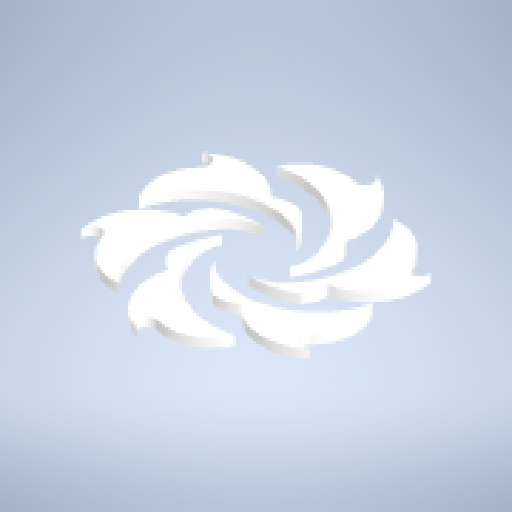
# Autodesk Inventor part: LOGO
Saved by Autodesk Inventor 2026.1 (Build 301233020, 233B)
## iProperties
Created: 2025-07-18
Part Number: LOGO
Material: 一般
Document SubType Name: Modeling
Designer: hibik
Density: 1 g/cm^3
Appearance: 既定
Author: hibik
Autodesk Inventor part; units mm, degrees
ref_plane "YZ Plane" through (0, 0, 0) normal (1, 0, 0) x (0, 1, 0)
ref_plane "XZ Plane" through (0, 0, 0) normal (0, 1, 0) x (-1, 0, 0)
sketch "スケッチ1" plane through (0, 0, 0) normal (0, 1, 0) x (-1, 0, 0)
  circle A0 centre (0, 0) radius 10 construction
  arc A1 (-2.5126, 0.5238) -> (1.9563, -1.6615) centre (0, 0) ccw
  arc A2 (-2.5126, 0.5238) -> (5.8099, -5.8825) centre (3.1979, -0.6667) ccw
  arc A3 (1.9563, -1.6615) -> (5.8099, -5.8825) centre (1.7789, -5.6931) ccw
  arc A4 (0.8333, -8.2275) -> (0.4466, -9.5023) centre (0.6667, -8.873) ccw
  arc A5 (1.9421, -1.6781) -> (4.7391, -6.2927) centre (1.6667, -5) ccw
  arc A6 (-3.2246, -3.3333) -> (-2.633, -0.5) centre (-0.9333, -2.3333) ccw
  arc A7 (-2.3333, -0.2667) -> (-2.3857, -2.355) centre (0.8049, -1.3903) ccw
  arc A8 (-2.3333, -0.2667) -> (-3.2246, -3.3333) centre (2.442, -3.3174) ccw
  point P0 (-2.091, -4.5491)
  point P1 (6.6984, -142.534)
  point P2 (12.5, -123.4123)
  point P3 (71.0869, -94.3908)
  point P4 (-0.885, -4.8329)
  point P5 (-1.6554, -4.7268)
  point P6 (-1.5359, -4.0754)
  point P7 (-39.4956, -7.5004)
  point P8 (87.1485, -88.2381)
  point P9 (1.4768, -1.669)
  point P10 (-1.7561, -3.7466)
  point P11 (1.1339, -1.7095)
  point P12 (1.4776, -1.672)
  point P13 (-2.5333, -0.4124)
  point P14 (-0.5469, -2.5077)
  point P15 (63.4693, -48.0608)
  point P16 (-2.4617, -0.7266)
  point P17 (-2.5059, -0.5553)
  point P18 (-2.6339, -0.7983)
  point P19 (-36.7334, -7.086)
  point P20 (-37.6897, 7.8571)
  point P21 (-35.7696, -6.328)
  point P22 (1.5501, -2.0457)
  point P23 (-0.6623, -2.4798)
  dimension "d0" = 20
  dimension "d1" = 5.1333
  dimension "d7" = 1.3333
  dimension "d9" = 1.6667
  dimension "d10" = 5
  dimension "d11" = 6.6667
  dimension "d13" = 5
  dimension "d15" = 2.3333
  dimension "d16" = 0.9333
  dimension "d17" = 0.6667
  dimension "d18" = 0.6667
  dimension "d19" = 11.6667
  dimension "d20" = 2.3333
  dimension "d21" = 0.2667
  dimension "d23" = 1
  dimension "d24" = 5.6667
  dimension "d25" = 3.3333
  constraints: 22 point on circle, 9 centre point, 6 tangent, 2 coincident
  measures "d0" diameter of A0
  measures "d1" diameter of A1
  measures "d7" diameter of A4
  measures "d9" horizontal distance of point (0, 0) A5.centre
  measures "d10" vertical distance of point (0, 0) A5.centre
  measures "d11" diameter of A5
  measures "d13" diameter of A6
  measures "d15" vertical distance of point (0, 0) A6.centre
  measures "d16" horizontal distance of point (0, 0) A6.centre
  measures "d17" vertical distance of point (0, 0) A2.centre
  measures "d18" horizontal distance of point (0, 0) A4.centre
  measures "d19" diameter of A2
  measures "d20" horizontal distance of point (0, 0) A7.start
  measures "d21" vertical distance of A7.start point (0, 0)
  measures "d23" vertical distance of A6.centre A6.start
  measures "d24" radius of A8
  measures "d25" radius of A7
extrude "押し出し1" add sketch "スケッチ1" along normal blind 0.6667 contours A6 A5 A2 | A2 A5 A6 | A5 A6 A3 A2 | A5 A4 A3 A6 | A8 A7 A1 | A1 A7 A2 A8 | A3 A6 A8 A2
pattern_circular "円形状パターン1" count 6 over 360 about axis through (0, -10, 0) along (0, 1, 0) of "押し出し1"
sketch "スケッチ2" plane through (1.0216, 0.6667, 3.1028) normal (0, 1, 0) x (0.9998, 0, -0.0187)
  line L0 (-2.4619, 1.0376) -> (-3.5173, 3.3772)
  line L1 (-3.5173, 3.3772) -> (-2.0188, 5.461)
  line L2 (-2.0188, 5.461) -> (0.5351, 5.2052)
  line L3 (0.5351, 5.2052) -> (1.5905, 2.8656)
  line L4 (1.5905, 2.8656) -> (0.092, 0.7817)
  line L5 (0.092, 0.7817) -> (-2.4619, 1.0376)
  circle A0 centre (-0.9634, 3.1214) radius 2.5667
  point P0 (-1.9392, 0.9852)
  point P1 (-3.3013, 2.8984)
  point P2 (-2.3254, 5.0346)
  point P3 (0.0125, 5.2576)
  point P4 (1.3745, 3.3443)
  point P5 (0.3987, 1.2082)
  dimension "d27" = 5.1333
  constraints: 12 end point, 2 coincident, 1 point on line, 16 other
ref_plane "作業平面1" through (1.099, 0.6667, 2.3195) normal (0.081, 0, -0.9967) x (-0.9967, 0, -0.081)
